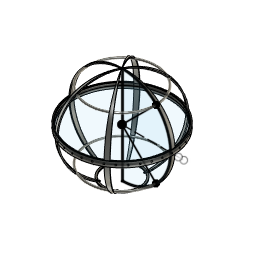
2022_10_01_Drone Soccer Invalide Ball With Led v1 (Autodesk Fusion 360 design; units mm, degrees)
Autodesk Fusion 360 part; units mm, degrees
note: some values were not read from the file. Set by a fixed rule: which sketch regions a step uses.
sketch "Sketch1" plane through (0, 0, 0) normal (0, 0, 1) x (1, 0, 0)
  circle A0 centre (0, 0) radius 97.5
  circle A1 centre (0, 0) radius 95
  dimension "d1" = 195
  dimension "d2" = 190
  constraint coincident A0.centre A1.centre
  constraint concentric A0 A1
  measures "d1" diameter of A0
  measures "d2" diameter of A1
sketch "Sketch2" plane through (0, 0, 0) normal (0, 1, 0) x (1, 0, 0)
  circle A0 centre (0, 0) radius 1.5
  dimension "d3" = 3
  constraint coincident A0.centre origin
  measures "d3" diameter of A0
extrude "Extrude1" add sketch "Sketch2" along normal blind 4 makes body 1
extrude "Extrude2" add sketch "Sketch1" along normal blind 5 and the other way blind 5 separate body makes body 2
move_body "Move1" bodies 1 to x (1, 0, 0) y (0, 1, 0) z (0, 0, 1) at (0, 96, 0)
pattern_circular "C-Pattern1" count 36 over 360 about axis through (0, 0, 1.75) along (0, 0, 1) of bodies 1 makes body 3 at (-15.4319, 96.1138, 0.1494) makes body 4 at (-33.7108, 92.7291, -1.4995) makes body 5 at (-47.3741, 85.0394, 0.1494) makes body 6 at (-63.3931, 75.6071, -1.4995) makes body 7 at (-74.9451, 64.182, -1.1247) makes body 8 at (-83.5469, 49.9592, 0.1494) makes body 9 at (-92.7035, 33.7811, -1.4995) makes body 10 at (-95.5954, 18.3716, 0.1494) makes body 11 at (-97.3333, 1.4925, 0.1494) makes body 12 at (-96.1138, -15.4319, 0.1494) makes body 13 at (-92.7291, -33.7108, -1.4995) makes body 14 at (-85.0394, -47.3741, 0.1494) makes body 15 at (-75.6071, -63.3931, 1.4995) makes body 16 at (-63.4504, -75.559, -1.4995) makes body 17 at (-49.9592, -83.5469, 0.1494) makes body 18 at (-33.7811, -92.7035, -1.4995) makes body 19 at (-16.271, -97.3197, -1.2179) makes body 20 at (-1.4925, -97.3333, 0.1494) makes body 21 at (15.4319, -96.1138, 0.1494) makes body 22 at (33.7108, -92.7291, -1.4995) makes body 23 at (48.0359, -86.1969, 0.0748) makes body 24 at (63.3931, -75.6071, 1.4995) makes body 25 at (75.559, -63.4504, -1.4995) makes body 26 at (84.891, -47.6312, 0.9057) makes body 27 at (91.8564, -32.2102, 0.9642) makes body 28 at (97.3197, -16.271, -1.2179) makes body 29 at (97.3333, -1.4925, 0.1494) makes body 30 at (96.1138, 15.4319, 0.1494) makes body 31 at (92.7291, 33.7108, -1.4995) makes body 32 at (86.1969, 48.0359, 0.0748) makes body 33 at (75.276, 63.7877, -1.4219) makes body 34 at (63.4504, 75.559, -1.4995) makes body 35 at (47.6312, 84.891, 0.9057) makes body 36 at (33.7811, 92.7035, -1.4995) makes body 37 at (16.271, 97.3197, -1.2179)
sketch "Sketch3" plane through (0, 0, 0) normal (0, 1, 0) x (1, 0, 0)
  line L0 (0, 0) -> (0, -97.5)
  line L1 (0, 97.5) -> (0, 0)
  arc A0 (0, -97.5) -> (0, 97.5) centre (0, 0) ccw
  line L2 (2, 0) -> (2, -95.4791)
  arc A1 (2, -95.4791) -> (2, 95.4791) centre (0, 0) ccw
  line L3 (2, 95.4791) -> (2, 0)
  line L4 (0, 0) -> (68.9429, -68.9429)
  line L5 (0, 0) -> (122.8535, 0) construction
  line L6 (0, 0) -> (68.9429, 68.9429)
  line L7 (0, 0) -> (112.0234, 0) construction
  circle A2 centre (67.5287, -67.5287) radius 2
  circle A3 centre (67.5287, 67.5287) radius 2
  line L8 (2, -95.4791) -> (0, -97.5)
  line L9 (2, 95.4791) -> (0, 97.5)
  dimension "d12" = 195
  dimension "d13" = -2
  dimension "d14" = 45
  dimension "d15" = 45
  constraint coincident L0.start L1.end
  constraint vertical L0
  constraint parallel L0 L1
  constraint horizontal L5
  constraint horizontal L7
  constraint coincident L4 A2.centre
  constraint coincident A1 A2.centre
  constraint tangent A0 A2
  constraint coincident L6 A3.centre
  constraint coincident A1 A3.centre
  constraint tangent A0 A3
  constraint coincident A0 L6.end
  constraint coincident A0 L4.end
  measures "d12" diameter of A0
  measures "d14" angle of L4 L5
  measures "d15" angle of L6 L7
sketch "Sketch4" plane through (0, 0, 0) normal (0, 1, 0) x (1, 0, 0)
copy_body "CopyPasteBodies1" bodies 2 makes body 38
move_body "Move2" bodies 38 to x (1, 0, 0) y (0, 1, 0) z (0, 0, 1) at (0, 0, 0)
combine "Combine1" operation add target body 37 tool bodies 25 7 28 32 8 17 26 24 33 34 13 2 30 36 1 22 31 16 35 3 15 27 23 9 11 14 29 12 5 6 18 10 19 4 20 21
scale "Scale1" factor 1.01 about (-95, 0, -5) bodies 38
move_body "Move3" bodies 38 to x (1, 0, 0) y (0, 1, 0) z (0, 0, 1) at (-0.7, 0, 0)
scale "Scale2" factor 0.99 about (0, 0, 0) bodies 37
extrude "Extrude3" cut sketch "Sketch1" along normal blind 90 and the other way blind 120 contours A1 bodies 37
revolve "Revolve1" add sketch "Sketch3" angle 5 about axis through (0, 0, 0) along (0, 0, 1) separate body contours A0 A1 A2 L8 | A0 A1 A3 L9 | A0 A1 A2 A3 makes body 39 at (62.5982, 3.0372, 74.6893)
pattern_circular "C-Pattern2" count 6 over 360 about axis through (0, 0, 0) along (0, 0, 1) of bodies 39 makes body 40 at (46.2604, 85.7953, -2.3203) makes body 41 at (-51.1707, 82.9604, -2.3203) makes body 42 at (-97.4312, -2.835, -2.3203) makes body 43 at (-46.2604, -85.7953, -2.3203) makes body 44 at (51.1707, -82.9604, -2.3203)
revolve "Revolve2" add sketch "Sketch3" angle 360 about axis through (0, 0, 0) along (0, 0, 1) contours A1 L4 A2 | A1 L4 A2 | A1 L6 A3 | A1 L6 A3 | A1 L4 A2 | A1 L4 A2 | A1 L6 A3 | A1 L6 A3 bodies 39 40 41 42 43 44
sketch "Sketch5" plane through (0, 0, 0) normal (0, 1, 0) x (1, 0, 0)
  line L0 (-100, 100) -> (100, 100)
  line L1 (100, 100) -> (100, 90)
  line L2 (100, 90) -> (-100, 90)
  line L3 (-100, 90) -> (-100, 100)
  dimension "d26" = 10
  constraint horizontal L0
  constraint vertical L1
  constraint horizontal L2
  constraint vertical L3
  measures "d26" distance of L0.start L2.end
extrude "Extrude4" cut sketch "Sketch5" along normal blind 140 and the other way blind 110 bodies 39
sketch "Sketch6" plane through (0, 0, 0) normal (0, 0, 1) x (1, 0, 0)
  circle A0 centre (0, 0) radius 38.0132
  circle A1 centre (0, 0) radius 34.8855
  constraint coincident A0.centre A1.centre
extrude "Extrude5" add sketch "Sketch6" along normal blind 2 separate body makes body 45
move_body "Move4" bodies 45 to x (1, 0, 0) y (0, 1, 0) z (0, 0, 1) at (0, 0, -91)
combine "Combine2" operation add target body 45 tool bodies 39 38
named bodies: "LedMesh", "HorizontalBorer", "ProtectBody"
